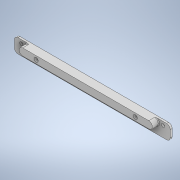
# Autodesk Inventor part: DisplayHolderUpper
Saved by Autodesk Inventor 2022 (Build 260153000, 153)
## iProperties
Created: 2021-04-23
Part Number: DisplayHolderUpper
Material: Generic
Document SubType Name: Modeling
Designer: Viktor
Density: 1 g/cm^3
Appearance: Default
Author: Viktor
## iProperties of the stored document DisplayHolderUpper_3DPrint.ipt
Created: 2021-04-23
Part Number: DisplayHolderUpper_3DPrint
Material: Generic
Document SubType Name: Modeling
Designer: Viktor
Density: 1 g/cm^3
Appearance: Default
Author: Viktor
Autodesk Inventor part; units mm, degrees
ref_plane "YZ Plane" through (0, 0, 0) normal (1, 0, 0) x (0, 1, 0)
ref_plane "XZ Plane" through (0, 0, 0) normal (0, 1, 0) x (-1, 0, 0)
ref_plane "XY Plane" through (0, 0, 0) normal (0, 0, 1) x (1, 0, 0)
sketch "Sketch7" plane through (0, 0, 0) normal (0, 0, 1) x (1, 0, 0)
  line L0 (-110, -10) -> (110, -10)
  line L1 (110, -10) -> (110, 10)
  line L2 (110, 10) -> (-110, 10)
  line L3 (-110, 10) -> (-110, -10)
  line L4 (-110, -10) -> (110, 10) construction
  line L5 (110, -10) -> (-110, 10) construction
  point P0 (0, 0)
  dimension "d27" = 20
  dimension "d28" = 220
  constraints: 12 end point, 2 midpoint, 2 parallel, 1 horizontal, 1 perpendicular
  measures "d27" distance of L2.end L0.start
  measures "d28" distance between parallel lines of L1 L3
extrude "Extrusion6" add sketch "Sketch7" along normal blind 2.8
sketch "Sketch8" plane through (0, 0, 2.8) normal (0, 0, 1) x (1, 0, 0)
  line L0 (-110, 10) -> (-110, -10) projected
  line L1 (-110, 0) -> (110, 0)
  line L2 (110, 0) -> (110, 10)
  line L3 (110, 10) -> (-110, 10)
  line L4 (-110, 10) -> (-110, 0)
  point P0 (0, 0)
  dimension "d32" = 10
  constraints: 8 end point, 2 parallel, 1 coincident, 1 horizontal, 1 midpoint, 1 perpendicular
  measures "d32" distance between parallel lines of L3 L1
extrude "Extrusion7" add sketch "Sketch8" along normal blind 9.2
sketch "Sketch9" plane through (0, 0, 12) normal (0, 0, 1) x (1, 0, 0)
  circle A0 centre (-70, 5) radius 2.85
  line L0 (0, 14) -> (0, -14) projected
  circle A1 centre (70, 5) radius 2.85
  line L1 (110, 10) -> (-110, 10) projected
  point P0 (0, 0)
  dimension "d35" = 5.7
  dimension "d36" = 5
  dimension "d37" = 70
  constraints: 2 centre point, 1 symmetric about line, 1 other
  measures "d35" diameter of A0
  measures "d36" distance from line of L1 A0.centre
  measures "d37" distance from line of L0 A0.centre
extrude "Extrusion8" cut sketch "Sketch9" against normal through all
fillet "Fillet4" radius 5 6 edges at (-110, 0, 7.4) (-110, 10, 6) (-110, -10, 1.4) (110, -10, 1.4) (110, 0, 7.4) (110, 10, 6)
sketch "Sketch10" plane through (0, 0, 12) normal (0, 0, 1) x (1, 0, 0)
  circle A0 centre (-100, 5) radius 2.3
  circle A1 centre (-70, 5) radius 2.85 projected
  line L0 (105, 10) -> (-105, 10) projected
  line L1 (0, 14) -> (0, -14) projected
  circle A2 centre (100, 5) radius 2.3
  point P0 (0, 0)
  dimension "d43" = 4.6
  dimension "d44" = 100
  dimension "d45" = 5
  dimension "d46" = 5
  constraints: 2 centre point, 1 symmetric about line, 1 other
  measures "d43" diameter of A0
  measures "d44" horizontal distance of point (0, 0) A0.centre
  measures "d45" distance from line of L0 A1.centre
  measures "d46" distance from line of L0 A0.centre
extrude "Extrusion9" cut sketch "Sketch10" against normal through all contours A0 | A2
sketch "Sketch11" plane through (0, 0, 12) normal (0, 0, 1) x (1, 0, 0)
  line L0 (-115, 10) -> (-94, 10)
  line L1 (-94, 10) -> (-94, -3.6473)
  line L2 (-94, -3.6473) -> (-115, -3.6473)
  line L3 (-115, -3.6473) -> (-115, 10)
  line L4 (-110, 5) -> (-110, -5) projected
  line L5 (-105, 0) -> (105, 0) projected
  line L6 (105, 10) -> (-105, 10) projected
  line L7 (0, 14) -> (0, -14) projected
  line L8 (115, 10) -> (94, 10)
  line L9 (94, 10) -> (94, -3.6473)
  line L10 (94, -3.6473) -> (115, -3.6473)
  line L11 (115, -3.6473) -> (115, 10)
  line L12 (110, 1.6834) -> (110, -5)
  point P0 (0, 0)
  point P1 (-110, 1.6834)
  point P2 (94, 0)
  dimension "d49" = 16
  constraints: 18 end point, 5 symmetric about line, 2 parallel, 1 horizontal, 1 perpendicular, 1 point on line
  measures "d49" distance between parallel lines of L4 L1
extrude "Extrusion10" cut sketch "Sketch11" against normal up to surface (9.2 mm away) contours L0 L1 L2 L3 | L6 L8 L11 L10 L9
fillet "Fillet6" radius 5 4 edges at (-94, 0, 7.4) (-94, 10, 7.4) (94, 0, 7.4) (94, 10, 7.4)
fillet "Fillet7" radius 1 3 edges at (-92.5357, 1.4643, 2.8) (92.5357, 1.4643, 2.8) (0, 0, 2.8)
equation "\"d46\" = d45"
body "Solid2"
